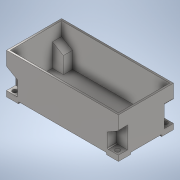
# Autodesk Inventor part: МПСТ Корпус
Saved by Autodesk Inventor 2022.1 (Build 261234020, 234B)
## iProperties
Created: 2021-11-18
Part Number: МПСТ Корпус
Material: Сталь, углеродистая
Document SubType Name: Modeling
Designer: Алексанян Г.
Density: 7.85 g/cm^3
Appearance: С умеренной полировкой
Author: Алексанян Г.
Autodesk Inventor part; units mm, degrees
ref_plane "YZ Plane" through (0, 0, 0) normal (1, 0, 0) x (0, 1, 0)
ref_plane "XZ Plane" through (0, 0, 0) normal (0, 1, 0) x (-1, 0, 0)
ref_plane "XY Plane" through (0, 0, 0) normal (0, 0, 1) x (1, 0, 0)
sketch "Эскиз1" plane through (0, 0, 0) normal (0, 1, 0) x (-1, 0, 0)
  line L0 (305, -150) -> (-305, -150)
  line L1 (-305, -150) -> (-305, 150)
  line L2 (-305, 150) -> (305, 150)
  line L3 (305, 150) -> (305, -150)
  line L4 (305, -150) -> (-305, 150) construction
  line L5 (-305, -150) -> (305, 150) construction
  point P0 (0, 0)
  dimension "d0" = 610
  dimension "d1" = 300
  constraints: 12 end point, 2 midpoint, 2 parallel, 1 horizontal, 1 perpendicular
  measures "d0" distance of L1.end L2.end
  measures "d1" distance of L0.end L1.end
extrude "Выдавливание1" add sketch "Эскиз1" against normal blind 220
sketch "Эскиз2" plane through (-305, 0, 150) normal (0, 0, 1) x (1, 0, 0)
  line L0 (65, -210) -> (545, -210)
  line L1 (545, -210) -> (545, -230)
  line L2 (545, -230) -> (65, -230)
  line L3 (65, -230) -> (65, -210)
  line L4 (610, -220) -> (0, -220) projected
  line L5 (65, -210) -> (545, -230) construction
  line L6 (545, -210) -> (65, -230) construction
  point P0 (305, 0)
  point P1 (305, -220)
  dimension "d4" = 480
  dimension "d5" = 20
  constraints: 12 end point, 3 midpoint, 2 parallel, 1 horizontal, 1 perpendicular
  measures "d4" distance of L1.end L2.end
  measures "d5" distance of L0.end L1.end
extrude "Выдавливание2" cut sketch "Эскиз2" against normal through all
sketch "Эскиз3" plane through (305, 0, 150) normal (1, 0, 0) x (0, 0, -1)
  line L0 (65, -210) -> (235, -210)
  line L1 (235, -210) -> (235, -230)
  line L2 (235, -230) -> (65, -230)
  line L3 (65, -230) -> (65, -210)
  line L4 (0, -220) -> (300, -220) projected
  line L5 (65, -210) -> (235, -230) construction
  line L6 (235, -210) -> (65, -230) construction
  point P0 (150, 0)
  point P1 (150, -220)
  dimension "d8" = 170
  dimension "d9" = 20
  constraints: 12 end point, 3 midpoint, 2 parallel, 1 horizontal, 1 perpendicular
  measures "d8" distance of L1.end L2.end
  measures "d9" distance of L0.end L1.end
extrude "Выдавливание3" cut sketch "Эскиз3" against normal through all
sketch "Эскиз4" plane through (-305, 0, 150) normal (0, 0, 1) x (1, 0, 0)
  line L0 (610, 0) -> (610, -220) projected
  line L1 (610, -190) -> (550, -190)
  line L2 (550, -190) -> (550, -110)
  line L3 (610, -110) -> (610, -190)
  line L4 (550, -110) -> (610, -75.359)
  line L5 (550, -110) -> (619.282, -110) construction
  line L6 (610, -220) -> (545, -220) projected
  point P0 (305, 0)
  point P1 (580, -190)
  dimension "d12" = 30
  dimension "d13" = 30
  dimension "d14" = 60
  dimension "d15" = 80
  constraints: 10 end point, 2 horizontal, 2 point on line, 1 equal length, 1 midpoint, 1 parallel, 1 perpendicular
  measures "d12" angle of L5 L4
  measures "d13" distance from line of L6 point (580, -190)
  measures "d14" distance between parallel lines of L2 L0
  measures "d15" distance from line of L1 L2.end
extrude "Выдавливание4" cut sketch "Эскиз4" against normal blind 50
sketch "Эскиз5" plane through (245, -190, 150) normal (0, 1, 0) x (1, 0, 0)
  line L0 (60, 50) -> (60, 0) projected
  line L1 (60, 0) -> (0, 0) projected
  point P0 (-245, 150)
  point P1 (35, 20)
  dimension "d18" = 25
  dimension "d19" = 20
  measures "d18" distance from line of L0 point (35, 20)
  measures "d19" distance from line of L1 point (35, 20)
hole "Отверстие1" at (280, -190, 130) direction (0, -1, 0) diameter 25 end through all
mirror "Зеркальное отражение1" about plane through (0, 0, 0) normal (1, 0, 0) of "Выдавливание4", "Отверстие1"
mirror "Зеркальное отражение2" about plane through (0, 0, 0) normal (0, 0, 1) of "Выдавливание4", "Отверстие1", "Зеркальное отражение1"
sketch "Эскиз6" plane through (0, 0, 0) normal (0, 1, 0) x (1, 0, 0)
  line L0 (-305, -150) -> (305, -150) construction
  line L1 (305, -150) -> (305, 150) construction
  line L2 (305, 150) -> (-305, 150) construction
  line L3 (-305, 150) -> (-305, -150) construction
  line L4 (-295, 140) -> (295, 140)
  line L5 (295, 140) -> (295, -140)
  line L6 (295, -140) -> (-295, -140)
  line L7 (-295, -140) -> (-295, 140)
  point P0 (0, 0)
  dimension "d27" = 10
  constraints: 8 end point, 3 other
  measures "d27" distance between parallel lines of L2 L4
extrude "Выдавливание5" cut sketch "Эскиз6" against normal up to surface (75.359 mm away)
sketch "Эскиз7" plane through (295, 0, 140) normal (0, 0, -1) x (-1, 0, 0)
  line L0 (50, -110) -> (-10, -75.359) construction
  line L1 (590, -75.359) -> (0, -75.359) projected
  line L2 (0, -75.359) -> (60, -110)
  line L3 (50, -110) -> (50, -190) projected
  line L4 (295, 70.8163) -> (295, -268.4276) construction
  line L5 (590, -75.359) -> (530, -110)
  line L6 (540, -190) -> (540, -110) projected
  line L7 (530, -110) -> (60, -110)
  point P0 (295, 0)
  dimension "d30" = 10
  dimension "d31" = 10
  constraints: 8 end point, 1 horizontal, 1 parallel, 1 symmetric about line, 1 vertical
  measures "d30" distance of L0.start L2.end
  measures "d31" distance from line of L6 L5.end
extrude "Выдавливание6" cut sketch "Эскиз7" along normal up to surface (280 mm away)
sketch "Эскиз8" plane through (-235, -110, 140) normal (0, 1, 0) x (1, 0, 0)
  line L0 (0, 280) -> (470, 280) construction
  line L1 (0, 0) -> (0, 280) construction
  line L2 (470, 0) -> (0, 0) construction
  line L3 (470, 0) -> (470, 280) construction
  line L4 (530, 50) -> (530, 230)
  line L5 (470, 0) -> (470, 280) projected
  line L6 (0, 280) -> (470, 280) projected
  line L7 (470, 280) -> (0, 280)
  line L8 (0, 0) -> (0, 280) projected
  line L9 (530, 50) -> (470, 50)
  line L10 (470, 50) -> (470, 0)
  line L11 (470, 0) -> (0, 0) projected
  line L12 (470, 0) -> (0, 0)
  line L13 (0, 0) -> (0, 50)
  line L14 (0, 50) -> (-60, 50)
  line L15 (-60, 50) -> (-60, 230)
  line L16 (235, -84.6684) -> (235, 409.964) construction
  line L17 (530, 230) -> (470, 230)
  line L18 (470, 230) -> (470, 280)
  line L19 (-60, 230) -> (0, 230)
  line L20 (0, 280) -> (0, 230)
  line L21 (-70, 40) -> (-10, 40) projected
  line L22 (-70, 225) -> (-70, 55) projected
  line L23 (-70, 240) -> (-10, 240) projected
  point P0 (235, 140)
  dimension "d37" = 10
  dimension "d38" = 10
  dimension "d39" = 10
  constraints: 26 end point, 7 point on line, 4 collinear, 4 perpendicular, 1 horizontal, 1 vertical, 3 other
  measures "d37" distance between parallel lines of L14 L21
  measures "d38" distance between parallel lines of L22 L15
  measures "d39" distance between parallel lines of L23 L19
extrude "Выдавливание7" cut sketch "Эскиз8" along normal mid plane 180
fillet "Сопряжение1" radius 5 20 edges at (-245, -110, 125) (-240, -210, 117.5) (-240, -210, -117.5) (240, -210, 117.5) (240, -210, -117.5) (245, -110, 125) (245, -110, -125) (-245, -110, -125) (272.5, -210, -85) (-272.5, -210, -85) (-272.5, -210, 85) (272.5, -210, 85) (305, -75.359, 125) (305, -75.359, -125) (-305, -75.359, -125) (-305, -75.359, 125) (-245, -190, 125) (245, -190, 125) (245, -190, -125) (-245, -190, -125)
equation "\"d38\" = d37"
equation "\"d39\" = d38"
